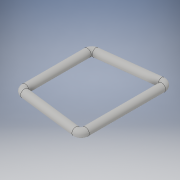
# Autodesk Inventor part: PKWS1-PIN
Saved by Autodesk Inventor 2019 (Build 230136000, 136)
## iProperties
Created: 2024-01-04
Part Number: PKWS1-PIN
Material: Generic
Catalog Web Link: www.cadenas.de
Description: PKWS-PIN-Snap Locks
Vendor: MISUMI
Document SubType Name: Modeling
Designer: psAdmin
Manufacturer: MISUMI
Mass: 0.0972013 g
Surface Area: 2.59203 cm^2
Volume: 0.0972013 cm^3
Density: 1 g/cm^3
Appearance: PSOLRGB-175-175-175
Category: PARTsolutions
Company: MISUMI
Title: PKWS1-PIN
Author: Cadenas PARTsolutions
Comments: Snap Locks
PSOL_IDENT_0: {$CADENAS_DATA/23d-libs/misumi/metric/44_handles_hinges/pkws_pin.prj},160 {VTYP=3D},{NB=PKWS1-PIN},{
PSOL_IDENT_1: LINA=PKWS1-PIN},{NN=PKWS-PIN},{DATE=04.06.2021 03:58:35},{GEOMDATE=17.02.2014 00:00:00},{VERSION=},{
PSOL_IDENT_2: LINEID=10},{WBVAR=},{WBNUMERIC=}  {NB=PKWS1-PIN},{LINA=PKWS1-PIN},{KT=DUMMY},{PN=PKWS1},{NO=1},{TL=4
PSOL_IDENT_3: 9 (5)},{MASS=11},{PPATH=assemblies_pkws\\pkws_templ.prj},{ANGLE=10.015},{X=8.000},{Y=4.000},{R=0.750
PSOL_IDENT_4: },{THICK=1.000},{Z=2.25},{DIST=21},{ANG=9.93658},{W=12.8435},{XZ=13.039095}
NB: PKWS1-PIN
NN: PKWS-PIN
NT: Snap Locks
NBSYN: $PN.-PIN
LINA: PKWS1-PIN
CATALOG: Misumi
PN: PKWS1
NO: 1
TL: 49 (5)
MASS: 11
ANGLE: 10.015
X: 8
Y: 4
R: 0.75
THICK: 1
DIST: 21
SUPPLIER: MISUMI
ARTICLENO: PKWS1-PIN
BOMINFO: PKWS1-PIN
CREATOR: CADENAS GmbH
Autodesk Inventor part; units mm, degrees
sketch "Sketch_1" plane through (0, 0, 0) normal (0, 0, 1) x (1, 0, 0)
  circle A0 centre (8, 0) radius 0.75
  constraints: 1 centre point
extrude "Extrusion1" add sketch "Sketch_1" along normal mid plane 14.8
sketch "Sketch_2" plane through (8, 0, -7.4) normal (0, 0, -1) x (-1, 0, 0)
  line L0 (0.85, 0.75) -> (0.85, -0.75)
  circle A0 centre (0, 0) radius 0.75
  constraints: 2 end point, 1 centre point
revolve "Revolution1" add sketch "Sketch_2" angle 97 about axis through (7.15, 0.75, -7.4) along (0, 1, 0)
sketch "Sketch_3" plane through (8, 0, 7.4) normal (0, 0, 1) x (1, 0, 0)
  line L0 (-0.85, -0.75) -> (-0.85, 0.75)
  circle A0 centre (0, 0) radius 0.75
  constraints: 2 end point, 1 centre point
revolve "Revolution2" add sketch "Sketch_3" angle 97 about axis through (7.15, -0.75, 7.4) along (0, -1, 0)
sketch "Sketch_8" plane through (0, 0, 0) normal (0, 0, 1) x (1, 0, 0)
  circle A0 centre (-5.0391, 0) radius 0.75
  constraints: 1 centre point
sketch "Sketch_4" plane through (7.0464, 0, -8.2437) normal (-0.9925462, 0, 0.1218693) x (0.1218693, 0, 0.9925462)
  circle A0 centre (0, 0) radius 0.75
  constraints: 1 centre point
extrude "Extrusion2" add sketch "Sketch_4" along normal blind 11.4243
sketch "Sketch_5" plane through (7.0464, 0, 8.2437) normal (-0.9925462, 0, -0.1218693) x (-0.1218693, 0, 0.9925462)
  circle A0 centre (0, 0) radius 0.75
  constraints: 1 centre point
extrude "Extrusion3" add sketch "Sketch_5" along normal blind 11.4243
sketch "Sketch_6" plane through (-4.2927, 0, -6.8514) normal (-0.9925462, 0, 0.1218693) x (0.1218693, 0, 0.9925462)
  line L0 (0.85, 0.75) -> (0.85, -0.75)
  circle A0 centre (0, 0) radius 0.75
  constraints: 2 end point, 1 centre point
revolve "Revolution3" add sketch "Sketch_6" angle 83 about axis through (-4.1891, 0.75, -6.0077) along (0, 1, 0)
sketch "Sketch_7" plane through (-4.2927, 0, 6.8514) normal (-0.9925462, 0, -0.1218693) x (-0.1218693, 0, 0.9925462)
  line L0 (-0.85, -0.75) -> (-0.85, 0.75)
  circle A0 centre (0, 0) radius 0.75
  constraints: 2 end point, 1 centre point
revolve "Revolution4" add sketch "Sketch_7" angle 83 about axis through (-4.1891, -0.75, 6.0077) along (0, -1, 0)
extrude "Extrusion4" add sketch "Sketch_8" along normal mid plane 12.0155
ref_plane "B_XY" through (8, 0, 0) normal (0, 0, 1) x (1, 0, 0)
ref_plane "B_YZ" through (8, 0, 0) normal (1, 0, 0) x (0, 1, 0)
ref_plane "B_ZX" through (8, 0, 0) normal (0, 1, 0) x (0, 0, 1)
ref_plane "C_XY" through (-5.0391, 0, 0) normal (0, 0, 1) x (1, 0, 0)
ref_plane "C_YZ" through (-5.0391, 0, 0) normal (1, 0, 0) x (0, 1, 0)
ref_plane "C_ZX" through (-5.0391, 0, 0) normal (0, 1, 0) x (0, 0, 1)
body "Solid1"
